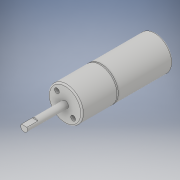
# Autodesk Inventor part: platform_motor
Saved by Autodesk Inventor 2019 (Build 230136000, 136)
## iProperties
Created: 2020-06-10
Part Number: platform_motor
Material: Generic
Document SubType Name: Modeling
Designer: Jorge
Density: 1 g/cm^3
Appearance: Default
Author: Jorge
Autodesk Inventor part; units mm, degrees
ref_plane "YZ Plane" through (0, 0, 0) normal (1, 0, 0) x (0, 1, 0)
ref_plane "XZ Plane" through (0, 0, 0) normal (0, 1, 0) x (-1, 0, 0)
ref_plane "XY Plane" through (0, 0, 0) normal (0, 0, 1) x (1, 0, 0)
sketch "Sketch1" plane through (0, 0, 0) normal (0, 0, 1) x (1, 0, 0)
  circle A0 centre (0, 0) radius 12.5
  dimension "d0" = 25
  constraints: 1 centre point, 1 coincident
  measures "d0" diameter of A0
extrude "Extrusion1" add sketch "Sketch1" along normal blind 26.5
fillet "Fillet1" radius 1 2 edges at (-12.5, 0, 26.5) (-12.5, 0, 0)
sketch "Sketch2" plane through (0, 0, 26.5) normal (0, 0, 1) x (1, 0, 0)
  circle A0 centre (-5.9291, 5.7365) radius 1.75
  line L0 (-5.9291, 5.7365) -> (0, 0) construction
  line L1 (0, 0) -> (5.9291, -5.7365) construction
  circle A1 centre (5.9291, -5.7365) radius 1.75
  dimension "d5" = 3.5
  dimension "d6" = 3.5
  dimension "d7" = 16.5
  constraints: 4 end point, 2 centre point, 2 collinear, 1 coincident
  measures "d5" diameter of A0
  measures "d6" diameter of A1
  measures "d7" distance of L0.start L1.end
extrude "Extrusion2" cut sketch "Sketch2" against normal blind 10
sketch "Sketch3" plane through (0, 0, 0) normal (0, 0, -1) x (-1, 0, 0)
  circle A0 centre (0, 0) radius 12.45
  dimension "d10" = 24.9
  constraints: 1 centre point, 1 coincident
  measures "d10" diameter of A0
extrude "Extrusion3" add sketch "Sketch3" along normal blind 40
sketch "Sketch4" plane through (0, 0, 26.5) normal (0, 0, 1) x (1, 0, 0)
  circle A0 centre (0, 0) radius 2.5
  dimension "d13" = 5
  constraints: 1 centre point, 1 coincident
  measures "d13" diameter of A0
extrude "Extrusion4" add sketch "Sketch4" along normal blind 30
sketch "Sketch5" plane through (0, 0, 56.5) normal (0, 0, 1) x (1, 0, 0)
  circle A0 centre (0, 0) radius 2.5 projected
  line L0 (-2.0152, 1.4796) -> (2.0152, 1.4796)
  arc A1 (2.0152, 1.4796) -> (-2.0152, 1.4796) centre (0, 0) ccw
  constraints: 4 point on circle, 2 end point, 1 centre point, 1 horizontal
extrude "Extrusion5" cut sketch "Sketch5" against normal blind 8 contours L0 A0 picked at (0.5388, 1.6221)
fillet "Fillet2" radius 1 1 edges at (12.45, 0, -40)
body "Solid1"
